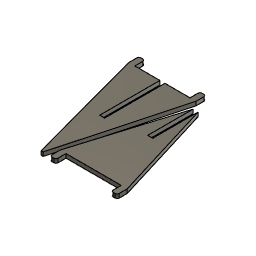
Gemüsehalter (Autodesk Fusion 360 design; units mm, degrees)
Autodesk Fusion 360 part; units mm, degrees
sketch "Skizze1" plane through (0, 0, 0) normal (0, 1, 0) x (1, 0, 0)
  line L0 (-27.5, 0) -> (0, 0)
  line L1 (0, 0) -> (0, -120)
  line L2 (0, -120) -> (-1, -120)
  line L3 (-1, -120) -> (-33.5, 0)
  line L4 (-33.5, 0) -> (-33.5, 10)
  line L5 (-33.5, 10) -> (-27.5, 10)
  line L6 (-27.5, 10) -> (-27.5, 0)
  line L7 (0, 0) -> (-2.5, 0)
  line L8 (-2.5, 0) -> (-2.5, -60)
  line L9 (-2.5, -60) -> (0, -60)
  line L10 (0, -60) -> (0, 0)
  line L11 (2.5, -60) -> (0, -60)
  line L12 (0, 0) -> (2.5, 0)
  line L13 (0, -120) -> (1, -120)
  line L14 (33.5, 0) -> (33.5, 10)
  line L15 (33.5, 10) -> (27.5, 10)
  line L16 (2.5, 0) -> (2.5, -60)
  line L17 (0, 0) -> (0, -120)
  line L18 (27.5, 10) -> (27.5, 0)
  line L19 (1, -120) -> (33.5, 0)
  line L20 (27.5, 0) -> (0, 0)
  line L21 (7.8524, -120) -> (7.8524, -110)
  line L22 (7.8524, -120) -> (13.8524, -120)
  line L23 (13.8524, -120) -> (13.8524, -110)
  line L24 (13.8524, -110) -> (41.3524, -110)
  line L25 (41.3524, -110) -> (41.3524, 0)
  line L26 (41.3524, 0) -> (7.8524, -110)
  line L27 (41.3524, -53.5) -> (38.8524, -53.5)
  line L28 (38.8524, -53.5) -> (38.8524, -8.209)
  line L29 (41.3524, 0) -> (74.8524, -110)
  line L30 (74.8524, -120) -> (74.8524, -110)
  line L31 (74.8524, -120) -> (68.8524, -120)
  line L32 (68.8524, -120) -> (68.8524, -110)
  line L33 (68.8524, -110) -> (41.3524, -110)
  line L34 (43.8524, -53.5) -> (43.8524, -8.209)
  line L35 (41.3524, -53.5) -> (43.8524, -53.5)
  dimension "d1" = 6
  dimension "d3" = 1
  dimension "d5" = 10
  dimension "d6" = 60
  dimension "d7" = 2.5
  dimension "d15" = 56.5
  dimension "d20" = 4
  dimension "d22" = 120
  dimension "d25" = 55
  constraint coincident L0.end L1.start
  constraint horizontal L0
  constraint perpendicular L0 L1
  constraint perpendicular L1 L2
  constraint perpendicular L2 L4
  constraint perpendicular L4 L5
  constraint perpendicular L0 L6
  constraint coincident L0 L3.end
  constraint horizontal L7
  constraint vertical L8
  constraint horizontal L9
  constraint vertical L10
  constraint symmetric L0.end L10 L1.start
  constraint symmetric L0.start L10 L18.end
  constraint symmetric L1.end L10 L2.start
  constraint symmetric L2.end L10 L13.end
  constraint symmetric L3.end L10 L14.start
  constraint symmetric L4.end L10 L14.end
  constraint symmetric L5.end L10 L15.end
  constraint symmetric L7.end L10 L12.end
  constraint symmetric L8.end L10 L11.start
  constraint symmetric L9.end L10 L11.end
  constraint parallel L17 L21
  constraint perpendicular L21 L22
  constraint perpendicular L22 L23
  constraint perpendicular L23 L24
  constraint perpendicular L24 L25
  constraint coincident L25 L27.start
  constraint perpendicular L25 L27
  constraint coincident L26 L28.end
  constraint perpendicular L27 L28
  constraint equal L9 L27
  constraint equal L6 L23
  constraint equal L0 L24
  constraint equal L4 L21
  constraint equal L5 L22
  constraint horizontal L0.end L25.end
  constraint symmetric L21.start L25 L30.start
  constraint symmetric L21.end L25 L29.end
  constraint symmetric L22.end L25 L31.end
  constraint symmetric L23.end L25 L32.end
  constraint symmetric L24.end L25 L33.end
  constraint symmetric L26.start L25 L29.start
  constraint symmetric L25 L27.start L35.start
  constraint symmetric L25 L27.end L34.start
  constraint symmetric L25 L28.end L34.end
  constraint collinear L13 L22
  measures "d1" distance of L4.end L5.end
  measures "d3" distance of L1.end L2.end
  measures "d5" distance of L0.end L5
  measures "d6" distance of L7.end L8.end
  measures "d7" distance of L1 L8
  measures "d15" distance of L24 L27
  measures "d20" distance of L19 L21.end
  measures "d22" distance of L0.end L1.end
  measures "d25" distance of L6 L18
extrude "Extrusion1" add sketch "Skizze1" along normal blind 4 contours L0 L1 L2 L3 L4 L5 L6 L8 L9 L17 | L1 L11 L13 L14 L15 L16 L17 L18 L19 L20 | L21 L22 L23 L24 L25 L26 L27 L28 | L25 L29 L30 L31 L32 L33 L34 L35 makes body 1 at (-10.8333, 0, 20) makes body 2 at (41.3524, 0, 91.1667)
fillet "Abrundung1" radius 2 8 edges at (33.5, 2, -10) (27.5, 2, -10) (-27.5, 2, -10) (-33.5, 2, -10) (7.8524, 2, 120) (13.8524, 2, 120) (68.8524, 2, 120) (74.8524, 2, 120) on bodies 1 2
equation "d6 = d22 / 2"
equation "d15 = d6 - 3.5 mm"
